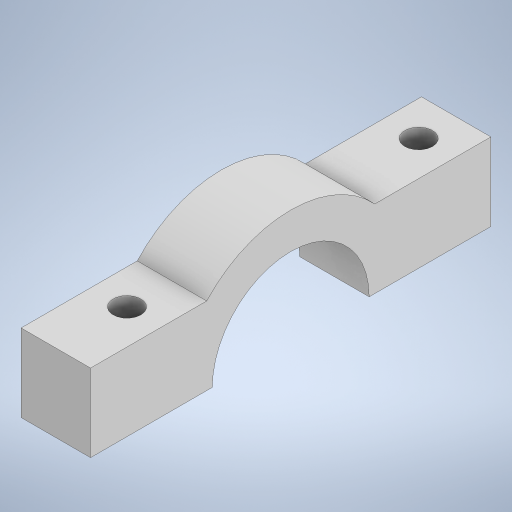
# Autodesk Inventor part: Lagerhalter1
Saved by Autodesk Inventor 2023 (Build 270158000, 158)
## iProperties
Created: 2022-05-03
Part Number: Lagerhalter1
Material: Generisch
Document SubType Name: Modeling
Designer: trist
Density: 1 g/cm^3
Appearance: Vorgabe
Author: trist
Autodesk Inventor part; units mm, degrees
ref_plane "YZ Plane" through (0, 0, 0) normal (1, 0, 0) x (0, 1, 0)
ref_plane "XZ Plane" through (0, 0, 0) normal (0, 1, 0) x (-1, 0, 0)
ref_plane "XY Plane" through (0, 0, 0) normal (0, 0, 1) x (1, 0, 0)
sketch "Skizze10" plane through (0, 0, 0) normal (1, 0, 0) x (0, 1, 0)
  arc A0 (0, -9.6) -> (0, 9.6) centre (0, 0) ccw
  line L0 (0, 0) -> (0, -24.5)
  line L1 (0, 0) -> (0, 24.5)
  line L2 (0, 15.79) -> (24.9524, 15.79) construction
  line L3 (-4.9905, 0) -> (29.9429, 0) projected
  line L4 (0, -19.91) -> (23.7326, -19.91) construction
  line L5 (0, 24.5) -> (9.5, 24.5)
  line L6 (9.5, 24.5) -> (9.5, 10.2835)
  arc A1 (9.5, -10.2835) -> (9.5, 10.2835) centre (0, 0) ccw
  line L7 (9.5, -10.2835) -> (9.5, -24.5)
  line L8 (0, -24.5) -> (9.5, -24.5)
  point P0 (0, 9.6)
  point P1 (9.5, -19.91)
  point P2 (9.5, 15.79)
  dimension "d79" = 9.6
  dimension "d80" = 24.5
  dimension "d81" = 24.5
  dimension "d82" = 15.79
  dimension "d83" = 19.91
  dimension "d84" = 9.5
  dimension "d85" = 14
  constraints: 16 end point, 6 point on line, 4 horizontal, 4 point on circle, 2 centre point, 2 coincident, 2 perpendicular, 2 vertical, 1 vertical alignment
  measures "d79" radius of A0
  measures "d80" distance of L0.start L0.end
  measures "d81" distance of L0.start L1.end
  measures "d82" distance between parallel lines of L2 L3
  measures "d83" distance between parallel lines of L3 L4
  measures "d84" distance of L0.end L7.end
  measures "d85" radius of A1
extrude "Extrusion9" add sketch "Skizze10" along normal mid plane 8.5 contours A0 L3 A1 L7 L8 L0 | A0 L1 L5 L6 A1 L3
sketch "Skizze11" plane through (0, 0, 0) normal (0, 1, 0) x (-1, 0, 0)
  circle A0 centre (0, -19.91) radius 1.7
  circle A1 centre (0, 15.79) radius 1.7
  line L0 (-4.25, -24.5) -> (-4.25, -10.2835) projected
  line L1 (0, -32.898) -> (0, 25.888) projected
  point P0 (0, 0)
  dimension "d88" = 15.79
  dimension "d89" = 19.91
  dimension "d90" = 3.4
  dimension "d91" = 3.4
  constraints: 2 centre point, 2 point on line
  measures "d88" distance of point (0, 0) A1.centre
  measures "d89" distance of point (0, 0) A0.centre
  measures "d90" diameter of A1
  measures "d91" diameter of A0
extrude "Extrusion10" cut sketch "Skizze11" along normal through all
sketch "Skizze12" plane through (0, 0, 0) normal (0, 1, 0) x (-1, 0, 0)
  line L0 (4.25, 9.6) -> (4.25, 24.5) projected
  line L1 (4.25, 23) -> (-1.05, 23)
  line L2 (-1.05, 23) -> (-1.05, 18.6)
  line L3 (-1.05, 18.6) -> (4.25, 18.6)
  line L4 (4.25, 18.6) -> (4.25, 23)
  line L5 (5.31, 0) -> (-2.11, 0) projected
  point P0 (0, 0)
  point P1 (4.25, 18.6)
  dimension "d94" = 4.4
  dimension "d95" = 5.3
  dimension "d96" = 18.6
  constraints: 8 end point, 2 parallel, 1 horizontal, 1 perpendicular, 1 point on line
  measures "d94" distance of L1.end L2.end
  measures "d95" distance of L1.start L1.end
  measures "d96" distance between parallel lines of L5 L3
extrude "Extrusion11" cut sketch "Skizze12" along normal blind 3.35
